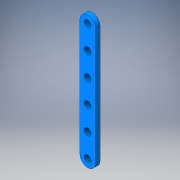
# Autodesk Inventor part: axlefixture
Saved by Autodesk Inventor 2016 (Build 200138000, 138)
## iProperties
Created: 2016-06-13
Part Number: axlefixture
Material: ABS Plastic
Document SubType Name: Modeling
Designer: hesaon
Density: 1.06 g/cm^3
Appearance: Smooth - White
Author: hesaon
Autodesk Inventor part; units mm, degrees
ref_plane "YZ Plane" through (0, 0, 0) normal (1, 0, 0) x (0, 1, 0)
ref_plane "XZ Plane" through (0, 0, 0) normal (0, 1, 0) x (-1, 0, 0)
ref_plane "XY Plane" through (0, 0, 0) normal (0, 0, 1) x (1, 0, 0)
sketch "Sketch1" plane through (0, 0, 0) normal (0, 1, 0) x (-1, 0, 0)
  line L0 (0, 52.5) -> (0, -52.5) construction
  line L1 (-7, 52.5) -> (-7, -52.5)
  line L2 (7, -52.5) -> (7, 52.5)
  arc A0 (7, 52.5) -> (-7, 52.5) centre (0, 52.5) ccw
  arc A1 (-7, -52.5) -> (7, -52.5) centre (0, -52.5) ccw
  circle A2 centre (0, 52.5) radius 3.1
  circle A3 centre (0, -52.5) radius 3.1
  circle A4 centre (0, 31.5) radius 3.1
  circle A5 centre (0, 10.5) radius 3.1
  circle A6 centre (0, -10.5) radius 3.1
  circle A7 centre (0, -31.5) radius 3.1
  point P0 (0, 0)
  point P1 (0, 0)
  dimension "d0" = 105
  dimension "d1" = 14
  dimension "d2" = 6.2
  dimension "d3" = 6.2
  dimension "d4" = 6.2
  dimension "d5" = 6.2
  dimension "d6" = 6.2
  dimension "d7" = 6.2
  dimension "d8" = 21
  dimension "d9" = 21
  dimension "d10" = 21
  dimension "d11" = 21
  dimension "d12" = 21
  constraints: 8 centre point, 8 end point, 4 point on circle, 4 point on line, 4 tangent, 3 coincident, 1 midpoint, 1 parallel, 1 vertical
  measures "d0" distance of L0.end L0.start
  measures "d1" distance between parallel lines of L1 L2
  measures "d2" diameter of A2
  measures "d3" diameter of A3
  measures "d4" diameter of A4
  measures "d5" diameter of A5
  measures "d6" diameter of A6
  measures "d7" diameter of A7
  measures "d8" distance of A4.centre A2.centre
  measures "d9" distance of A5.centre A4.centre
  measures "d10" distance of A6.centre A5.centre
  measures "d11" distance of A7.centre A6.centre
  measures "d12" distance of L0.end A7.centre
extrude "Extrusion1" add sketch "Sketch1" along normal blind 4
body "Solid1"
